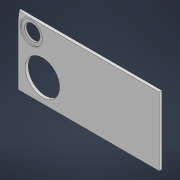
# Autodesk Inventor part: Front_L
Saved by Autodesk Inventor 2022 (Build 260153000, 153)
## iProperties
Created: 2022-04-08
Part Number: Front_L
Material: Типовые
Document SubType Name: Modeling
Designer: Kalugin_a
Density: 1 g/cm^3
Appearance: По умолчанию
Author: Kalugin_a
Autodesk Inventor part; units mm, degrees
ref_plane "YZ Plane" through (0, 0, 0) normal (1, 0, 0) x (0, 1, 0)
ref_plane "XZ Plane" through (0, 0, 0) normal (0, 1, 0) x (-1, 0, 0)
sketch "Front0" plane through (0, 0, 0) normal (0, 0, 1) x (1, 0, 0)
  line L0 (0, 0) -> (600, 0)
  line L1 (600, 0) -> (600, 290)
  line L2 (600, 290) -> (0, 290)
  line L3 (0, 290) -> (0, 0)
  circle A0 centre (104, 96) radius 73
  circle A1 centre (104, 96) radius 91
  circle A2 centre (57, 237) radius 47
  circle A3 centre (57, 237) radius 33
  line L4 (36, 290) -> (0, 250)
  line L5 (196, 290) -> (196, 0) construction
  point P0 (47.17, 0)
  point P1 (0, 87)
  dimension "d0" = 600
  dimension "d1" = 290
  dimension "d2" = 146
  dimension "d3" = 182
  dimension "d4" = 94
  dimension "d5" = 66
  dimension "d17" = 96
  dimension "d36" = 104
  dimension "d37" = 57
  dimension "d38" = 53
  dimension "d40" = 92
  dimension "d24" = 146
  dimension "d25" = 182
  constraints: 12 end point, 4 centre point, 4 coincident, 4 point on line, 2 parallel, 2 perpendicular, 1 horizontal
  measures "d0" distance of L2.end L1.end
  measures "d1" distance of L1.end L0.end
  measures "d2" diameter of A0
  measures "d3" diameter of A1
  measures "d4" diameter of A2
  measures "d5" diameter of A3
  measures "d17" distance from line of L0 A0.centre
  measures "d36" distance from line of L3 A1.centre
  measures "d37" distance from line of L3 A2.centre
  measures "d38" distance from line of L2 A2.centre
  measures "d40" distance from line of A0.centre L5
extrude "Выдавливание2" add sketch "Front0" against normal blind 12 contours L3 L4 L2 L1 L0 | L3 L2 L4 | A1 | A2
ref_plane "РабПлоскость9" through (0, 290, -6) normal (0.1626, -0.1464, -0.9758) x (0.9864, 0, 0.1644)
split "Разделение5" plane through (0, 290, -6) removes the side toward (-0.1626, 0.1464, 0.9758)
extrude "Выдавливание7" cut sketch "Front0" against normal blind 4 contours A2
